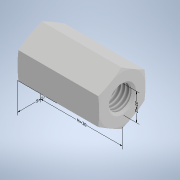
# Autodesk Inventor part: Hexagon nut DIN 6334 M10 51103.100.040(High)
Saved by Autodesk Inventor 2021 (Build 250183000, 183)
## iProperties
Created: 2025-04-05
Part Number: Hexagon nut DIN 6334 M10 51103.100.040(High)
Material: Generic
Catalog Web Link: www.cadenas.de
Description: DIN 6334-Hexagon extension nuts
Vendor: FABORY
Document SubType Name: Modeling
Designer: psAdmin
Manufacturer: FABORY
Mass: 56 g
Surface Area: 29.1056 cm^2
Volume: 5.83197 cm^3
Density: 1 g/cm^3
Appearance: PSOLRGB-175-175-175
Category: PARTsolutions
Company: FABORY
Title: Hexagon nut DIN 6334 M10
Author: Cadenas PARTsolutions
Comments: Hexagon extension nuts
PSOL_IDENT_0: {$CADENAS_DATA/23d-libs/fabory/3_nuts/din_6334.prj},232 {M=Nenngewinde},{VTYP=3D},{NB=Hexagon nut DI
PSOL_IDENT_1: N 6334 M10 51103.100.040(High)},{LINA=Hexagon nut DIN 6334 M10},{NN=DIN 6334},{DATE=13.02.2023 21:14
PSOL_IDENT_2: :46},{GEOMDATE=13.03.2019 09:47:48},{VERSION=},{LINEID=51570},{WBVAR=LOD},{WBNUMERIC=}  {NB=Sechskan
PSOL_IDENT_3: tmutter DIN 6334 M10 51103.100.040(High)},{LINA=Sechskantmutter DIN 6334 M10},{KT=DUMMY},{CNSORDERNO=
PSOL_IDENT_4: 51103.100.040},{NENNID=M10X40},{D=10.000},{BRAND=Fabory},{STANDARD=DIN 6334},{THREAD=Metric thread},
PSOL_IDENT_5: {THREADDIRECTIO=Right},{STYLE=},{TYPE=Hexagon connection nut},{BASICMATERIAL=Stainless steel},{GRADE=
PSOL_IDENT_6: A2},{SURFACETREATME=},{HEADSHAPE=},{DRIVINGFEATURE=Hexagon},{COLOR=},{CNSMASSEXACT=0.05600},{COMPARA
PSOL_IDENT_7: BLESTAN=},{ADDITIONALINFO=},{ROHS=Y},{APPROVAL=},{EANCODE=8715494537858},{INTRASTATCODE=73181630},{E
PSOL_IDENT_8: CLASS=23-11-08-08},{UNSPSC=31161727},{ETIM=EC002360},{URL=https://www.fabory.com/en-GB/p/51103100040
PSOL_IDENT_9: },{VARIANT=0},{PACKAGING=25},{FAB_NENN=M10},{FAB_GEO=Diameter (d)=M10;m=30;P=1.5;s=17},{FAB_ARTICLEN
PSOL_IDENT_10: UMBER=51103.100.040},{FABNETWEIGHT=56.000},{NENN=M10},{D1=8.376},{P=1.500},{DIN962THREAD=},{XLH=0},{
PSOL_IDENT_11: DIN962OPT2=},{M=30},{S=17},{SWX=},{E=19.60},{SKD2=2.000},{OPTIONS2L='',' - ','din_962_std.jpg','-SK'
PSOL_IDENT_12: ,'SK Drahtloch','din_962_s_4.jpg'},{DIN962FTHREAD=0},{CNSAVOID=0},{DIST=15.666667},{LOD=High},{LINK1=
PSOL_IDENT_13: 51103},{LINK2=100},{LINK3=040},{INFOPATH=https://www.fabory.com/en-GB/p/51103100040},{STANDARDSMALL=
PSOL_IDENT_14: din_6334.png}
NB: Hexagon nut DIN 6334 M10 51103.100.040(High)
NN: DIN 6334
NT: Hexagon extension nuts
NBSYN: Hexagon nut DIN 6334 $NENN. $CNSORDERNO.($LOD.)
LINA: Hexagon nut DIN 6334 M10
CATALOG: Fabory
ROWDESC: M10
OFFICIAL_STANDARD_NUMBERS: DIN 6334
CNSORDERNO: 51103.100.040
NENNID: M10X40
D: 10
BRAND: Fabory
STANDARD: DIN 6334
THREAD: Metric thread
THREADDIRECTIO: Right
TYPE: Hexagon connection nut
BASICMATERIAL: Stainless steel
GRADE: A2
DRIVINGFEATURE: Hexagon
CNSMASSEXACT: 0.056
ROHS: Y
EANCODE: 8715494537858
INTRASTATCODE: 73181630
ECLASS: 23-11-08-08
UNSPSC: 31161727
ETIM: EC002360
URL: https://www.fabory.com/en-GB/p/51103100040
PACKAGING: 25
P: 1.5
M: 30
S: 17
E: 19.6
LOD: High
SUPPLIER: FABORY
ARTICLENO: Hexagon nut DIN 6334 M10 51103.100.040(High)
BOMINFO: Hexagon nut DIN 6334 M10
CREATOR: CADENAS GmbH
Autodesk Inventor part; units mm, degrees
sketch "Sketch_1" plane through (0, 0, 0) normal (0, 0, 1) x (1, 0, 0)
  line L0 (30, 0) -> (0, 0)
  line L1 (0, 0) -> (0, 10.2)
  line L2 (0, 10.2) -> (30, 10.2)
  line L3 (30, 10.2) -> (30, 0)
  line L4 (30, 0) -> (0, 0)
  constraints: 10 end point
revolve "Revolution1" add sketch "Sketch_1" angle 360 about axis through (30, 0, 0) along (-1, 0, 0)
sketch "Sketch_4" plane through (0, 0, 0) normal (0, 0, 1) x (1, 0, 0)
  line L0 (30, 0) -> (0, 0)
  line L1 (0, 8.5) -> (0.4555, 10.2)
  line L2 (0.4555, 10.2) -> (0, 10.2)
  line L3 (0, 10.2) -> (0, 8.5)
  constraints: 8 end point
revolve "Revolution2" cut sketch "Sketch_4" angle 360 about axis through (30, 0, 0) along (1, 0, 0)
sketch "Sketch_5" plane through (0, 0, 0) normal (0, 0, 1) x (1, 0, 0)
  line L0 (30, 0) -> (0, 0)
  line L1 (29.5445, 10.2) -> (30, 8.5)
  line L2 (30, 8.5) -> (30, 10.2)
  line L3 (30, 10.2) -> (29.5445, 10.2)
  constraints: 8 end point
revolve "Revolution3" cut sketch "Sketch_5" angle 360 about axis through (30, 0, 0) along (1, 0, 0)
sketch "Sketch_3" plane through (0, 0, 0) normal (0, 0, 1) x (1, 0, 0)
  line L0 (30, 0) -> (0, 0)
  line L1 (0, 0) -> (0, 5)
  line L2 (0, 5) -> (0.812, 4.188)
  line L3 (0.812, 4.188) -> (29.188, 4.188)
  line L4 (29.188, 4.188) -> (30, 5)
  line L5 (30, 5) -> (30, 0)
  line L6 (30, 0) -> (0, 0)
  constraints: 14 end point
revolve "Revolution4" cut sketch "Sketch_3" angle 360 about axis through (30, 0, 0) along (1, 0, 0)
thread "Thread1" size "M10x1.5" class "6H" standard "ISO Metric profile" full length
sketch "Sketch_2" plane through (0, 0, 0) normal (1, 0, 0) x (0, 1, 0)
  line L0 (34, 34) -> (-34, 34)
  line L1 (-34, 34) -> (-34, -34)
  line L2 (-34, -34) -> (34, -34)
  line L3 (34, -34) -> (34, 34)
  line L4 (-4.9075, 8.5) -> (-9.815, 0)
  line L5 (-9.815, 0) -> (-4.9075, -8.5)
  line L6 (-4.9075, -8.5) -> (4.9075, -8.5)
  line L7 (4.9075, -8.5) -> (9.815, 0)
  line L8 (9.815, 0) -> (4.9075, 8.5)
  line L9 (4.9075, 8.5) -> (-4.9075, 8.5)
  constraints: 20 end point
extrude "Extrusion1" cut sketch "Sketch_2" along normal mid plane 62
ref_plane "IP1_XY" through (0, 0, 0) normal (1, 0, 0) x (0, 0, -1)
ref_plane "IP1_YZ" through (0, 0, 0) normal (0, 0, -1) x (0, 1, 0)
ref_plane "IP1_ZX" through (0, 0, 0) normal (0, 1, 0) x (1, 0, 0)
ref_plane "IP2_XY" through (30, 0, 0) normal (1, 0, 0) x (0, 0, -1)
ref_plane "IP2_YZ" through (30, 0, 0) normal (0, 0, -1) x (0, 1, 0)
ref_plane "IP2_ZX" through (30, 0, 0) normal (0, 1, 0) x (1, 0, 0)
body "Solid1"
